Autodesk Fusion 360 part; units mm, degrees
(part 2 of 2)
sketch "Skizze18" plane through (0, 0, 43) normal (0, 0, 1) x (-1, 0, 0)
  line L0 (-20.1786, -58.75) -> (-85.1607, -58.75)
  line L1 (-85.1607, -58.75) -> (-89.8214, -55)
  line L2 (-89.8214, -55) -> (-85.1607, -51.25)
  line L3 (-85.1607, -51.25) -> (-20.1786, -51.25)
  line L4 (-20.1786, -51.25) -> (-20.1786, -58.75)
  spline S0 degree 3 poles (-101.2424, -56.0053) (-101.4993, -55.8834) (-101.9991, -55.6463) (-102.344, -55.2145) (-102.5117, -55.0046) knots 0 0 0 0 0.084034 0.16353 0.16353 0.16353 0.16353
  spline S1 degree 3 poles (-102.5117, -55.0046) (-102.6393, -54.6353) (-102.9898, -53.6205) (-102.9694, -52.5411) (-102.9565, -51.8545) knots 0 0 0 0 0.116519 0.320189 0.320189 0.320189 0.320189
  spline S2 degree 3 poles (-102.9565, -51.8545) (-102.9544, -51.3248) (-102.9508, -50.4155) (-102.7064, -49.5416) (-102.6044, -49.177) knots 0 0 0 0 0.157982 0.271128 0.271128 0.271128 0.271128
  spline S3 degree 3 poles (-102.6044, -49.177) (-102.45, -48.8976) (-102.1215, -48.3033) (-101.5409, -47.9478) (-101.2332, -47.7594) knots 0 0 0 0 0.094114 0.200246 0.200246 0.200246 0.200246
  spline S4 degree 3 poles (-101.2332, -47.7594) (-100.8403, -47.6004) (-99.9658, -47.2465) (-99.0206, -47.2247) (-98.5, -47.2128) knots 0 0 0 0 0.126135 0.28077 0.28077 0.28077 0.28077
  spline S5 degree 3 poles (-98.5, -47.2128) (-97.995, -47.2238) (-97.0815, -47.2438) (-96.2371, -47.5873) (-95.8595, -47.7409) knots 0 0 0 0 0.14998 0.271283 0.271283 0.271283 0.271283
  spline S6 degree 3 poles (-95.8595, -47.7409) (-95.5608, -47.9257) (-94.9838, -48.2827) (-94.6307, -48.861) (-94.4605, -49.1399) knots 0 0 0 0 0.103727 0.200337 0.200337 0.200337 0.200337
  spline S7 degree 3 poles (-94.4605, -49.1399) (-94.3399, -49.524) (-94.0444, -50.4652) (-94.0438, -51.4544) (-94.0435, -52.0398) knots 0 0 0 0 0.120183 0.294445 0.294445 0.294445 0.294445
  spline S8 degree 3 poles (-94.0435, -52.0398) (-94.0493, -52.4647) (-94.0601, -53.2574) (-94.188, -54.0395) (-94.2474, -54.4024) knots 0 0 0 0 0.127264 0.237425 0.237425 0.237425 0.237425
  spline S9 degree 3 poles (-94.2474, -54.4024) (-94.3653, -54.7245) (-94.6159, -55.4089) (-95.2352, -55.7988) (-95.563, -56.0053) knots 0 0 0 0 0.100073 0.212645 0.212645 0.212645 0.212645
  spline S10 degree 3 poles (-95.563, -56.0053) (-95.345, -56.134) (-94.904, -56.3945) (-94.6463, -56.8374) (-94.5161, -57.0615) knots 0 0 0 0 0.074612 0.15095 0.15095 0.15095 0.15095
  spline S11 degree 3 poles (-94.5161, -57.0615) (-94.4163, -57.3351) (-94.1984, -57.9326) (-94.1821, -58.5694) (-94.1733, -58.9145) knots 0 0 0 0 0.086816 0.189552 0.189552 0.189552 0.189552
  spline S12 degree 3 poles (-94.1733, -58.9145) (-94.2011, -59.503) (-94.2526, -60.5897) (-94.9351, -61.4294) (-95.248, -61.8144) knots 0 0 0 0 0.171436 0.316557 0.316557 0.316557 0.316557
  spline S13 degree 3 poles (-95.248, -61.8144) (-95.6821, -62.0973) (-96.6536, -62.7304) (-97.8186, -62.767) (-98.4629, -62.7872) knots 0 0 0 0 0.152673 0.341629 0.341629 0.341629 0.341629
  spline S14 degree 3 poles (-98.4629, -62.7872) (-99.1861, -62.7788) (-100.4361, -62.7643) (-101.4531, -62.0569) (-101.8817, -61.7588) knots 0 0 0 0 0.210731 0.364237 0.364237 0.364237 0.364237
  spline S15 degree 3 poles (-101.8817, -61.7588) (-102.1568, -61.3559) (-102.7586, -60.4744) (-102.8028, -59.4033) (-102.8267, -58.8218) knots 0 0 0 0 0.143562 0.314061 0.314061 0.314061 0.314061
  spline S16 degree 3 poles (-102.8267, -58.8218) (-102.8252, -58.4686) (-102.8225, -57.8643) (-102.603, -57.3037) (-102.5117, -57.0707) knots 0 0 0 0 0.104759 0.17925 0.17925 0.17925 0.17925
  spline S17 degree 3 poles (-102.5117, -57.0707) (-102.3638, -56.8823) (-102.0165, -56.4403) (-101.5247, -56.1639) (-101.2424, -56.0053) knots 0 0 0 0 0.07123 0.167142 0.167142 0.167142 0.167142
  line L5 (-14.664, -62.5) -> (-14.664, -47.5)
  line L6 (-14.664, -47.5) -> (-10.9209, -47.5)
  line L7 (-10.9209, -47.5) -> (-10.9209, -55.542)
  spline S18 degree 3 poles (-10.9209, -55.542) (-10.9254, -56.0074) (-10.9322, -56.7072) (-10.8613, -57.4029) (-10.8376, -57.6359) knots 0 0 0 0 0.139453 0.209683 0.209683 0.209683 0.209683
  spline S19 degree 3 poles (-10.8376, -57.6359) (-10.7949, -57.747) (-10.7058, -57.9792) (-10.4879, -58.1007) (-10.3743, -58.164) knots 0 0 0 0 0.034599 0.072268 0.072268 0.072268 0.072268
  spline S20 degree 3 poles (-10.3743, -58.164) (-10.1745, -58.2172) (-9.6299, -58.3621) (-9.0645, -58.3543) (-8.7066, -58.3493) knots 0 0 0 0 0.061805 0.168453 0.168453 0.168453 0.168453
  line L8 (-8.7066, -58.3493) -> (-8.336, -58.3493)
  line L9 (-8.336, -58.3493) -> (-8.336, -60.1004)
  spline S21 degree 3 poles (-8.336, -60.1004) (-9.1727, -60.3292) (-10.7638, -60.7644) (-11.9137, -61.9418) (-12.4589, -62.5) knots 0 0 0 0 0.254912 0.484769 0.484769 0.484769 0.484769
  line L10 (-12.4589, -62.5) -> (-14.664, -62.5)
  line L11 (-102.25, -45) -> (-102.25, -25.2285)
  line L12 (-102.25, -25.2285) -> (-94.75, -25.2285)
  line L13 (-94.75, -25.2285) -> (-94.75, -45)
  line L14 (-94.75, -45) -> (-102.25, -45)
  circle A0 centre (-96.95, -18.1) radius 2.5
  circle A1 centre (-96.95, -91.9) radius 2.5
  line L15 (-102.25, -65) -> (-94.75, -65)
  line L16 (-94.75, -65) -> (-94.75, -84.7715)
  line L17 (-94.75, -84.7715) -> (-102.25, -84.7715)
  line L18 (-102.25, -84.7715) -> (-102.25, -65)
  line L19 (-7.75, -65) -> (-7.75, -84.7715)
  line L20 (-7.75, -84.7715) -> (-15.25, -84.7715)
  line L21 (-15.25, -84.7715) -> (-15.25, -65)
  line L22 (-15.25, -65) -> (-7.75, -65)
  line L23 (-7.75, -45) -> (-15.25, -45)
  line L24 (-15.25, -45) -> (-15.25, -25.2285)
  line L25 (-15.25, -25.2285) -> (-7.75, -25.2285)
  line L26 (-7.75, -25.2285) -> (-7.75, -45)
  line L27 (-7.75, -10.9715) -> (-15.25, -10.9715)
  line L28 (-15.25, -10.9715) -> (-15.25, 0)
  line L29 (-15.25, 0) -> (-20.1786, 0)
  line L30 (-20.1786, 0) -> (-20.1786, -45)
  line L31 (-20.1786, -45) -> (-27.6786, -45)
  line L32 (-27.6786, -45) -> (-27.6786, 0)
  line L33 (-27.6786, 0) -> (-32.6071, 0)
  line L34 (-32.6071, 0) -> (-32.6071, -45)
  line L35 (-32.6071, -45) -> (-40.1071, -45)
  line L36 (-40.1071, -45) -> (-40.1071, 0)
  line L37 (-40.1071, 0) -> (-45.0357, 0)
  line L38 (-45.0357, 0) -> (-45.0357, -45)
  line L39 (-45.0357, -45) -> (-52.5357, -45)
  line L40 (-52.5357, -45) -> (-52.5357, 0)
  line L41 (-52.5357, 0) -> (-57.4643, 0)
  line L42 (-57.4643, 0) -> (-57.4643, -45)
  line L43 (-57.4643, -45) -> (-64.9643, -45)
  line L44 (-64.9643, -45) -> (-64.9643, 0)
  line L45 (-64.9643, 0) -> (-69.8929, 0)
  line L46 (-69.8929, 0) -> (-69.8929, -45)
  line L47 (-69.8929, -45) -> (-77.3929, -45)
  line L48 (-77.3929, -45) -> (-77.3929, 0)
  line L49 (-77.3929, 0) -> (-82.3214, 0)
  line L50 (-82.3214, 0) -> (-82.3214, -45)
  line L51 (-82.3214, -45) -> (-89.8214, -45)
  line L52 (-89.8214, -45) -> (-89.8214, 0)
  line L53 (-89.8214, 0) -> (-94.75, 0)
  line L54 (-94.75, 0) -> (-94.75, -10.9715)
  line L55 (-94.75, -10.9715) -> (-102.25, -10.9715)
  line L56 (-102.25, -10.9715) -> (-102.25, 0)
  line L57 (-102.25, 0) -> (-105, 0)
  arc A2 (-105, 0) -> (-110, -5) centre (-105, -5) ccw
  line L58 (-110, -5) -> (-110, -105)
  arc A3 (-110, -105) -> (-105, -110) centre (-105, -105) ccw
  line L59 (-105, -110) -> (-102.25, -110)
  line L60 (-102.25, -110) -> (-102.25, -99.0285)
  line L61 (-102.25, -99.0285) -> (-94.75, -99.0285)
  line L62 (-94.75, -99.0285) -> (-94.75, -110)
  line L63 (-94.75, -110) -> (-89.8214, -110)
  line L64 (-89.8214, -110) -> (-89.8214, -65)
  line L65 (-89.8214, -65) -> (-82.3214, -65)
  line L66 (-82.3214, -65) -> (-82.3214, -110)
  line L67 (-82.3214, -110) -> (-77.3929, -110)
  line L68 (-77.3929, -110) -> (-77.3929, -65)
  line L69 (-77.3929, -65) -> (-69.8929, -65)
  line L70 (-69.8929, -65) -> (-69.8929, -110)
  line L71 (-69.8929, -110) -> (-64.9643, -110)
  line L72 (-64.9643, -110) -> (-64.9643, -65)
  line L73 (-64.9643, -65) -> (-57.4643, -65)
  line L74 (-57.4643, -65) -> (-57.4643, -110)
  line L75 (-57.4643, -110) -> (-52.5357, -110)
  line L76 (-52.5357, -110) -> (-52.5357, -65)
  line L77 (-52.5357, -65) -> (-45.0357, -65)
  line L78 (-45.0357, -65) -> (-45.0357, -110)
  line L79 (-45.0357, -110) -> (-40.1071, -110)
  line L80 (-40.1071, -110) -> (-40.1071, -65)
  line L81 (-40.1071, -65) -> (-32.6071, -65)
  line L82 (-32.6071, -65) -> (-32.6071, -110)
  line L83 (-32.6071, -110) -> (-27.6786, -110)
  line L84 (-27.6786, -110) -> (-27.6786, -65)
  line L85 (-27.6786, -65) -> (-20.1786, -65)
  line L86 (-20.1786, -65) -> (-20.1786, -110)
  line L87 (-20.1786, -110) -> (-15.25, -110)
  line L88 (-15.25, -110) -> (-15.25, -99.0285)
  line L89 (-15.25, -99.0285) -> (-7.75, -99.0285)
  line L90 (-7.75, -99.0285) -> (-7.75, -110)
  line L91 (-7.75, -110) -> (-5, -110)
  arc A4 (-5, -110) -> (0, -105) centre (-5, -105) ccw
  line L92 (0, -105) -> (0, -5)
  arc A5 (0, -5) -> (-5, 0) centre (-5, -5) ccw
  line L93 (-5, 0) -> (-7.75, 0)
  line L94 (-7.75, 0) -> (-7.75, -10.9715)
  circle A6 centre (-13.05, -18.1) radius 2.5
  circle A7 centre (-13.05, -91.9) radius 2.5
  circle A8 centre (-13.05, -91.9) radius 1.5
  circle A9 centre (-13.05, -18.1) radius 1.5
  circle A10 centre (-96.95, -91.9) radius 1.5
  circle A11 centre (-96.95, -18.1) radius 1.5
  dimension "d121" = 3
  constraint concentric A7 A8
  measures "d121" diameter of A8
extrude "Extrusion18" add sketch "Skizze18" against normal blind 3 contours A0 | A1 | A6 | A7 bodies 2 4
split "Teilen2" by plane through (55, 55, 40) normal (0, 0, -1) bodies 2 makes body 5 at (68.5758, 43.0614, 39)
copy_body "Körper->Berechn1" bodies 5 removing the originals makes body 6 in component "Center"
copy_body "Körper->Berechn2" bodies 2 removing the originals makes body 7 in component "Top"
copy_body "Körper->Berechn3" bodies 1 removing the originals makes body 8 in component "Bottom"
component "Center" placed x (1, 0, 0) y (0, 1, 0) z (0, 0, 1) at (0, 0, 0)
component "Top" placed x (1, 0, 0) y (0, 1, 0) z (0, 0, 1) at (0, 0, 0)
component "Bottom" placed x (1, 0, 0) y (0, 1, 0) z (0, 0, 1) at (0, 0, 0)
equation "d9 = 5 mm + ( ( d12 / 2 mm ) * 1 ) * 1 mm + 1 mm"
equation "d15 = 90 mm - 13 m"
equation "d19 = 100 mm - 13 mm"
equation "d29 = ( d28 - d26 ) / 2"
equation "d31 = ( d30 - d27 ) / 2"
equation "d63 = 10 mm"
equation "d67 = d66"
equation "d68 = d67"
equation "d69 = d63"
equation "d70 = d69"
equation "d71 = d70"
equation "d98 = d97 / 2"
equation "d106 = d105 / 2"
equation "d107 = d106"
equation "d116 = ( 7.5 / 2 ) * 1 mm"
equation "d117 = d116"
